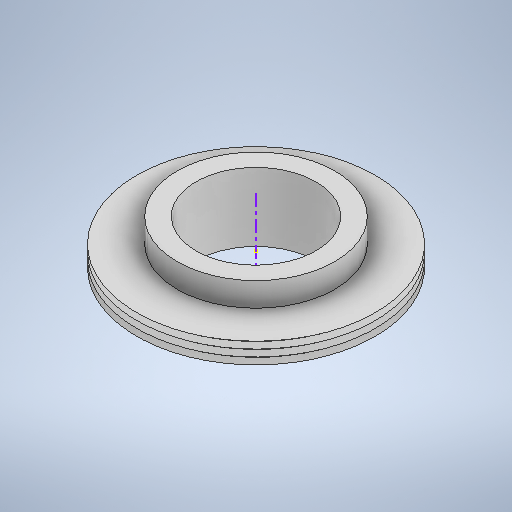
# Autodesk Inventor part: 34_Vong_chan_dau
Saved by Autodesk Inventor 2025.2 (Build 292293000, 293)
## iProperties
Created: 2024-11-26
Part Number: 34_Vong_chan_dau
Material: Generic
Document SubType Name: Modeling
Designer: hongquan
Density: 1 g/cm^3
Appearance: Default
Author: hongquan
Autodesk Inventor part; units mm, degrees
ref_plane "YZ Plane" through (0, 0, 0) normal (1, 0, 0) x (0, 1, 0)
ref_plane "XZ Plane" through (0, 0, 0) normal (0, 1, 0) x (-1, 0, 0)
ref_plane "XY Plane" through (0, 0, 0) normal (0, 0, 1) x (1, 0, 0)
sketch "Sketch1" plane through (0, 0, 0) normal (1, 0, 0) x (0, 1, 0)
  line L0 (10.3439, 0) -> (-10.3439, 0) construction
  line L1 (8.828, -17.5) -> (-11.172, -17.5)
  line L2 (8.828, -17.5) -> (8.828, -23)
  line L3 (8.828, -23) -> (1.828, -23)
  line L4 (1.828, -23) -> (1.828, -34.8153)
  line L5 (1.828, -34.8153) -> (-4.172, -34.8153)
  line L6 (-4.172, -34.8153) -> (-4.172, -23)
  line L7 (-4.172, -23) -> (-11.172, -23)
  line L8 (-11.172, -23) -> (-11.172, -17.5)
  line L9 (0, 48.9131) -> (0, -72.8322) construction
  point P0 (0, 0)
  point P1 (0, 0)
  dimension "d0" = 35
  dimension "d1" = 5.5
  dimension "d2" = 6
  dimension "d3" = 7
  constraints: 20 end point, 5 perpendicular, 4 horizontal, 3 vertical, 2 equal length, 1 coincident, 1 midpoint
  measures "d0" diameter of L1 L0
  measures "d1" distance of L1.start L2.end
  measures "d2" distance of L4.end L5.end
  measures "d3" distance of L2.end L3.end
revolve "Revolution1" add sketch "Sketch1" angle 360 about axis through (0, 10.3439, 0) along (0, -1, 0)
sketch "Sketch2" plane through (0, 0, 0) normal (1, 0, 0) x (0, 1, 0)
  line L0 (1.828, 34.8153) -> (1.828, -34.8153) projected
  line L1 (-4.172, 34.8153) -> (-4.172, -34.8153) projected
  line L2 (1.828, 34.8153) -> (1.828, -34.8153) projected
  line L3 (-4.172, 34.8153) -> (-4.172, -34.8153) projected
  line L4 (1.828, 34.8153) -> (1.828, -34.8153) projected
  line L5 (-4.172, 34.8153) -> (-4.172, -34.8153) projected
  line L6 (1.828, 34.8153) -> (1.828, -34.8153) construction
  line L7 (-4.172, 34.8153) -> (-4.172, -34.8153) construction
  line L8 (1.828, 34.8153) -> (1.828, -34.8153) construction
  line L9 (-4.172, 34.8153) -> (-4.172, -34.8153) construction
  line L10 (1.828, 34.8153) -> (1.828, -34.8153) construction
  line L11 (-4.172, 34.8153) -> (-4.172, -34.8153) construction
  line L12 (0.828, -33.5153) -> (1.828, -34.8153) construction
  line L13 (1.828, -34.8153) -> (-0.172, -34.8153) construction
  line L14 (-0.172, -34.8153) -> (0.828, -33.5153) construction
  line L15 (0.828, -34.8153) -> (0.828, -33.5153) construction
  line L16 (1.828, -34.8153) -> (-4.172, -34.8153) construction
  line L17 (0.828, -33.5153) -> (1.828, -34.8153)
  line L18 (-0.172, -34.8153) -> (1.828, -34.8153)
  line L19 (0.828, -33.5153) -> (-0.172, -34.8153)
  point P0 (0, 0)
  dimension "d5" = 1.3
  dimension "d6" = 2
  constraints: 14 end point, 2 collinear, 1 horizontal, 1 midpoint, 1 vertical, 1 other
  measures "d5" distance of L15.start L12.start
  measures "d6" distance of L0.end L13.end
sketch "Sketch3" plane through (0, 0, 0) normal (0, 0, 1) x (1, 0, 0)
  point P0 (0, 0)
sketch "Sketch4" plane through (0, 0, 0) normal (1, 0, 0) x (0, 1, 0)
  line L0 (14.7871, 0) -> (-17.2316, 0)
  point P0 (0, 0)
  constraints: 2 end point, 1 horizontal
revolve "Revolution2" cut sketch "Sketch2" angle 360 about axis through (0, 14.7871, 0) along (0, -1, 0)
pattern_linear "Rectangular Pattern1" count 4 spacing 2 along (0, -1, 0) of "Revolution2"
body "Solid1"
